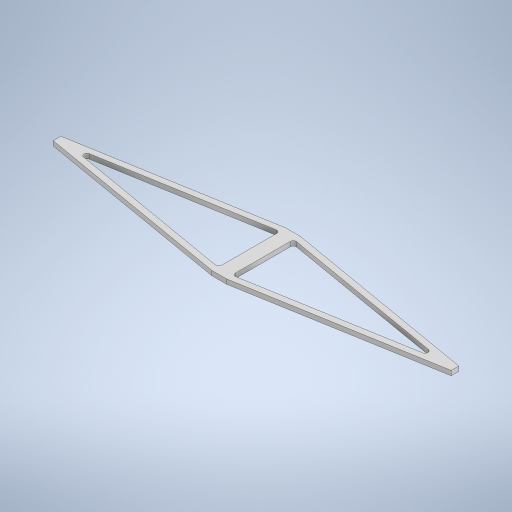
# Autodesk Inventor part: Main Support
Saved by Autodesk Inventor 2023 (Build 270158000, 158)
## iProperties
Created: 2023-03-16
Part Number: Main Support
Material: Generic
Document SubType Name: Modeling
Designer: bugme
Density: 1 g/cm^3
Appearance: Default
Author: bugme
Autodesk Inventor part; units mm, degrees
ref_plane "YZ Plane" through (0, 0, 0) normal (1, 0, 0) x (0, 1, 0)
ref_plane "XZ Plane" through (0, 0, 0) normal (0, 1, 0) x (-1, 0, 0)
ref_plane "XY Plane" through (0, 0, 0) normal (0, 0, 1) x (1, 0, 0)
sketch "Sketch1" plane through (0, 0, 0) normal (0, 1, 0) x (-1, 0, 0)
  line L0 (420, 0) -> (-420, 0) projected
  line L1 (0, 50) -> (-10, 50)
  line L2 (0, -50) -> (-10, -50)
  line L3 (-10, -50) -> (-270, -5.1724)
  line L4 (-270, 5.1724) -> (-10, 50)
  line L5 (0, 50) -> (0, -50)
  line L6 (0, 50) -> (10, 50)
  line L7 (0, -50) -> (10, -50)
  line L8 (10, -50) -> (270, -5.1724)
  line L9 (270, 5.1724) -> (10, 50)
  line L10 (-270, 0) -> (270, 0)
  line L11 (0, -70) -> (0, 70) projected
  line L12 (-270, 5.1724) -> (-270, -5.1724)
  line L13 (270, 5.1724) -> (270, -5.1724)
  line L14 (0, 42) -> (9.3154, 42)
  line L15 (9.3154, 42) -> (252.9154, 0)
  line L16 (252.9154, 0) -> (9.3154, -42)
  line L17 (9.3154, -42) -> (0, -42)
  line L18 (0, 42) -> (-9.3154, 42)
  line L19 (-9.3154, 42) -> (-252.9154, 0)
  line L20 (-252.9154, 0) -> (-9.3154, -42)
  line L21 (-9.3154, -42) -> (0, -42)
  line L22 (9.3154, 42) -> (9.3154, -42)
  line L23 (-9.3154, 42) -> (-9.3154, -42)
  point P0 (0, 0)
  point P1 (300, 0)
  point P2 (-300, 0)
  dimension "d36" = 600
  dimension "d38" = 10
  dimension "d39" = 100
  dimension "d42" = 540
  dimension "d44" = 8
  dimension "d45" = 8
  constraints: 44 end point, 5 symmetric about line, 4 vertical, 2 point on line, 1 horizontal, 1 parallel, 6 other
  measures "d36" distance of point (-300, 0) point (300, 0)
  measures "d38" distance of L1.start L1.end
  measures "d39" distance of L1.start L2.start
  measures "d42" distance of L10.start L10.end
  measures "d44" distance between parallel lines of L8 L16
  measures "d45" distance between parallel lines of L4 L19
extrude "Main_block" add sketch "Sketch1" along normal blind 6.35 contours L13 L8 L7 L5 L17 L16 L0 | L0 L15 L14 L5 L6 L9 L13 | L22 L17 L5 L0 | L0 L5 L14 L22 | L5 L21 L23 L0 | L0 L23 L18 L5 | L18 L19 L0 L12 L4 L1 L5 | L5 L2 L3 L12 L0 L20 L21
fillet "Fillet7" radius 4 6 edges at (-9.3154, 3.175, -42) (9.3154, 3.175, -42) (9.3154, 3.175, 42) (-9.3154, 3.175, 42) (252.9154, 3.175, 0) (-252.9154, 3.175, 0)
body "Solid1"
